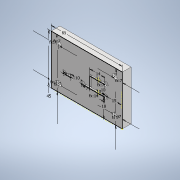
# Autodesk Inventor part: Millifluidic Board
Saved by Autodesk Inventor 2021 (Build 250183000, 183)
## iProperties
Created: 2020-06-06
Part Number: Millifluidic Board
Material: Generic
Document SubType Name: Modeling
Designer: natha
Density: 1 g/cm^3
Appearance: Default
Author: natha
Autodesk Inventor part; units mm, degrees
ref_plane "YZ Plane" through (0, 0, 0) normal (1, 0, 0) x (0, 1, 0)
ref_plane "XZ Plane" through (0, 0, 0) normal (0, 1, 0) x (-1, 0, 0)
sketch "points for corner holes and base plate" plane through (0, 0, 0) normal (0, 0, 1) x (1, 0, 0)
  line L0 (0, 0) -> (-65, 0)
  line L1 (-65, 0) -> (-65, 45)
  line L2 (-65, 45) -> (0, 45)
  line L3 (0, 45) -> (0, 0)
  point P0 (-7, 38)
  point P1 (-7, 7)
  point P2 (-58, 7)
  point P3 (-58, 38)
  dimension "d26" = 45
  dimension "d27" = 65
  dimension "d91" = 7
  dimension "d92" = 7
  dimension "d93" = 7
  dimension "d94" = 7
  dimension "d95" = 7
  dimension "d96" = 7
  dimension "d97" = 7
  dimension "d98" = 7
  constraints: 8 end point, 2 parallel, 1 horizontal, 1 perpendicular
  measures "d26" distance of L0.end L1.end
  measures "d27" distance of L1.end L2.end
  measures "d91" distance from line of L2 point (-7, 38)
  measures "d92" distance from line of L3 point (-7, 38)
  measures "d93" distance from line of L3 point (-7, 7)
  measures "d94" distance from line of L0 point (-7, 7)
  measures "d95" distance from line of L1 point (-58, 7)
  measures "d96" distance from line of L0 point (-58, 7)
  measures "d97" distance from line of L1 point (-58, 38)
  measures "d98" distance from line of L2 point (-58, 38)
extrude "Extrusion base plate" add sketch "points for corner holes and base plate" against normal blind 8
ref_plane "plane above base plate to create rib" through (0, 0, 1) normal (0, 0, 1) x (1, 0, 0)
sketch "channels and points for valves and for connectors" plane through (0, 0, 1) normal (0, 0, 1) x (1, 0, 0)
  line L0 (-36, 18) -> (-29, 18)
  line L1 (-29, 18) -> (-29, 28)
  line L2 (-29, 18) -> (-15, 18)
  line L3 (-46, 18) -> (-53, 18)
  line L4 (-29, 28) -> (-15, 28)
  line L5 (-60.6, 0) -> (-7.4, 0) construction
  line L6 (0, 30) -> (0, 16) construction
  point P0 (-22, 28)
  point P1 (-22, 18)
  dimension "d106" = 10
  dimension "d107" = 14
  dimension "d108" = 14
  dimension "d109" = 7
  dimension "d110" = 10
  dimension "d111" = 7
  dimension "d116" = 15
  dimension "d117" = 18
  dimension "d132" = 7
  dimension "d133" = 7
  constraints: 10 end point, 6 coincident, 3 point on line, 2 horizontal, 2 midpoint, 1 perpendicular
  measures "d106" distance between parallel lines of L4 L2
  measures "d107" distance of L1.end L4.end
  measures "d108" distance of L0.end L2.end
  measures "d109" distance of L0.start L0.end
  measures "d110" distance of L3.start L0.start
  measures "d111" distance of L3.start L3.end
  measures "d116" distance from line of L6 L2.end
  measures "d117" distance from line of L5 L2.end
  measures "d132" distance of L2.end point (-22, 18)
  measures "d133" distance of L4.end point (-22, 28)
rib "channels as rib" sketch "channels and points for valves and for connectors" thickness 1 direction (0, 0, -1) end up to next extend profile no curves L0 L1 L2 L3 L4
sketch "Sketch11" plane through (0, 0, 1) normal (0, 0, 1) x (1, 0, 0)
  line L0 (-15, 28.5) -> (-15, 27.5) projected
  line L1 (-29, 28.5) -> (-15, 28.5) projected
  line L2 (-29, 28) -> (-29, 28.5) projected
  line L3 (-29.5, 28) -> (-29, 28) projected
  line L4 (-29.5, 18.5) -> (-29.5, 28) projected
  line L5 (-36, 18.5) -> (-29.5, 18.5) projected
  line L6 (-36, 17.5) -> (-36, 18.5) projected
  line L7 (-15, 17.5) -> (-36, 17.5) projected
  line L8 (-15, 18.5) -> (-15, 17.5) projected
  line L9 (-28.5, 18.5) -> (-15, 18.5) projected
  line L10 (-28.5, 27.5) -> (-28.5, 18.5) projected
  line L11 (-15, 27.5) -> (-28.5, 27.5) projected
  line L12 (-53, 17.5) -> (-53, 18.5) projected
  line L13 (-46, 17.5) -> (-53, 17.5) projected
  line L14 (-46, 18.5) -> (-46, 17.5) projected
  line L15 (-53, 18.5) -> (-46, 18.5) projected
  line L16 (-29, 28) -> (-29.5, 28)
  line L17 (-29.5, 28) -> (-29.5, 28.5)
  line L18 (-29.5, 28.5) -> (-29, 28.5)
  line L19 (-29, 28.5) -> (-29, 28)
  line L20 (-29.5, 18.5) -> (-29.5, 28) projected
  line L21 (-29, 28.5) -> (-15, 28.5) projected
  point P0 (0, 0)
  constraints: 8 end point, 2 collinear, 2 parallel, 1 horizontal, 1 perpendicular
extrude "extrusion of rib to get cutout" cut sketch "Sketch11" against normal blind 2.3
sketch "Sketch6" plane through (0, 0, 0) normal (0, 0, 1) x (1, 0, 0)
  ellipse E0 centre (-22, 18) end of major axis (-19.5, 18) minor radius 1.75
  point P0 (0, 0)
  dimension "d58" = 2.5
  dimension "d59" = 1.75
  constraints: 1 centre point, 1 coincident, 1 other
extrude "valve space extrusion" cut sketch "Sketch6" against normal blind 1.3
sketch "Sketch7" plane through (0, 0, 0) normal (0, 0, 1) x (1, 0, 0)
  line L0 (-22.75, 16.25) -> (-21.25, 16.25)
  line L1 (-21.25, 16.25) -> (-21.25, 19.75)
  line L2 (-21.25, 19.75) -> (-22.75, 19.75)
  line L3 (-22.75, 19.75) -> (-22.75, 16.25)
  point P0 (0, 0)
  point P1 (-22, 18)
  dimension "d62" = 1.5
  dimension "d63" = 3.5
  dimension "d136" = 0.75
  dimension "d137" = 1.75
  constraints: 8 end point, 2 parallel, 1 horizontal, 1 perpendicular
  measures "d62" distance of L1.end L2.end
  measures "d63" distance of L2.end L0.start
  measures "d136" distance from line of L3 point (-22, 18)
  measures "d137" distance from line of L0 point (-22, 18)
extrude "valve bar extrusion" add sketch "Sketch7" against normal blind 2
sketch "Projected points for every valve" plane through (0, 0, 0) normal (0, 0, 1) x (1, 0, 0)
  point P0 (0, 0)
  point P1 (-22, 28)
  point P2 (-22, 18)
pattern_sketch "all valve spaces" of "valve space extrusion", "valve bar extrusion" from (-22, 18, 0) copies at (-22, 28, 0)
sketch "projected point for connector holes" plane through (0, 0, 0) normal (0, 0, 1) x (1, 0, 0)
  point P0 (0, 0)
  point P1 (-53, 18)
  point P2 (-46, 18)
  point P3 (-15, 18)
  point P4 (-15, 28)
  point P5 (-36, 18)
hole "holes for connectors" at (-36, 18, 0) at (-46, 18, 0) at (-53, 18, 0) at (-15, 18, 0) at (-15, 28, 0) direction (0, 0, -1) diameter 4.1 depth 1.3
hole "holes for corners" at (-58, 7, 0) at (-58, 38, 0) at (-7, 7, 0) at (-7, 38, 0) direction (0, 0, -1) diameter 4.5 end through all
body "Solid1"
